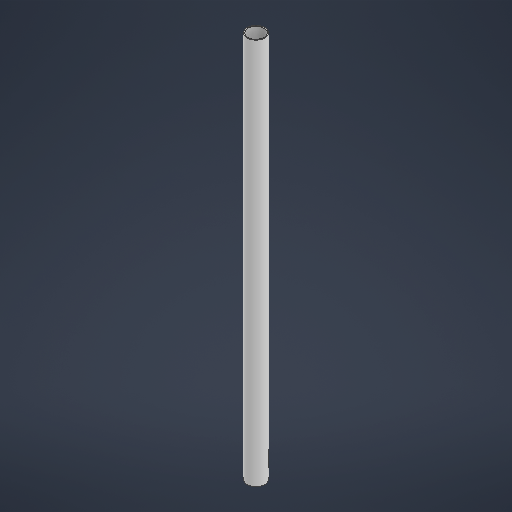
# Autodesk Inventor part: tubo cubierta tornillo
Saved by Autodesk Inventor 2026.1 (Build 301233020, 233B)
## iProperties
Created: 2025-12-03
Part Number: tubo cubierta tornillo
Material: Genérico
Document SubType Name: Modeling
Designer: benja
Density: 1 g/cm^3
Appearance: Valor por defecto
Author: benja
Autodesk Inventor part; units mm, degrees
ref_plane "YZ Plane" through (0, 0, 0) normal (1, 0, 0) x (0, 1, 0)
ref_plane "XZ Plane" through (0, 0, 0) normal (0, 1, 0) x (-1, 0, 0)
ref_plane "XY Plane" through (0, 0, 0) normal (0, 0, 1) x (1, 0, 0)
sketch "Boceto1" plane through (0, 0, 0) normal (0, 1, 0) x (-1, 0, 0)
  circle A0 centre (0, 0) radius 17.05
  circle A1 centre (0, 0) radius 19.05
  dimension "d0" = 34.1
  dimension "d1" = 38.1
  constraints: 2 centre point, 2 coincident
  measures "d0" diameter of A0
  measures "d1" diameter of A1
extrude "Extrusión1" add sketch "Boceto1" along normal blind 813.6
sketch "Boceto2" plane through (0, 0, 0) normal (0, 0, 1) x (1, 0, 0)
  line L0 (0, 0) -> (-263.1264, 0)
  line L1 (-263.1264, 0) -> (-263.1264, 271)
  line L2 (-263.1264, 135.5) -> (-17.2798, 135.5)
  line L3 (-19.05, 0) -> (-19.05, 813.6) projected
  line L4 (-17.2798, 135.5) -> (-17.2798, 51.5895)
  line L5 (-17.2798, 51.5895) -> (12.7202, 51.5895)
  line L6 (12.7202, 51.5895) -> (12.7202, 21.5895)
  line L7 (12.7202, 21.5895) -> (-17.2798, 21.5895)
  line L8 (-17.2798, 21.5895) -> (-17.2798, 51.5895)
  dimension "d4" = 271
  dimension "d5" = 30
  dimension "d6" = 30
  constraints: 16 end point, 4 perpendicular, 2 horizontal, 2 parallel, 1 midpoint
  measures "d4" distance of L0.end L1.end
  measures "d5" distance of L6.end L7.end
  measures "d6" distance of L5.end L6.end
extrude "Extrusión2" cut sketch "Boceto2" against normal blind 813.6 contours L5 L6 L7 L8
